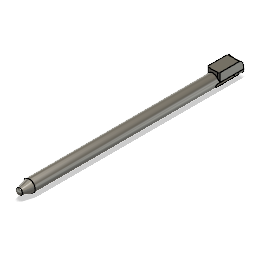
DSi Stylus v9 (Autodesk Fusion 360 design; units mm, degrees)
Autodesk Fusion 360 part; units mm, degrees
sketch "Sketch1" plane through (0, 0, 0) normal (0, 0, 1) x (1, 0, 0)
  circle A0 centre (0, 0) radius 2.5
  dimension "d1" = 5
  constraint coincident A0.centre origin
  measures "d1" diameter of A0
extrude "Extrude1" add sketch "Sketch1" along normal blind 92.2
chamfer "Chamfer1" distance 1.5 distance2 5 1 edges at (-2.3308, -0.904, 92.2) measured on face at (-0.8863, 0.2321, 92.2)
fillet "Fillet1" radius 1.3435 1 edges at (-0.9323, 0.3616, 92.2)
sketch "Sketch2" plane through (0, 0, 0) normal (1, 0, 0) x (0, 0, -1)
  line L0 (0, 0) -> (0, 3.6)
  line L1 (0, 3.6) -> (-10.8, 3.6)
  line L2 (-10.8, 3.6) -> (-10.8, 0)
  line L3 (-10.8, 0) -> (0, 0)
  line L4 (0, 0) -> (0, 3.6)
  dimension "d7" = 3.6
  dimension "d8" = 10.8
  constraint coincident L0.start L3.end
  constraint vertical L0
  constraint horizontal L1
  constraint vertical L2
  constraint horizontal L3
  constraint vertical L4
  measures "d7" distance of L0.start L0.end
  measures "d8" distance of L0.end L1.end
extrude "Extrude2" add sketch "Sketch2" along normal blind 2.5 and the other way blind 2.5
fillet "Fillet2" radius 0.5 1 edges at (2.5, 1.8, 10.8)
fillet "Fillet3" radius 0.5 1 edges at (-2.5, 1.8, 10.8)
sketch "Sketch3" plane through (-2.5, 0, 0) normal (-1, 0, 0) x (0, 0, 1)
  line L0 (10.3, 0) -> (10.3, 3.6)
  line L1 (10.3, 3.6) -> (0, 3.6)
  line L2 (0, 3.6) -> (0, 0)
  line L3 (0, 0) -> (10.3, 0)
  line L4 (0, 3.6) -> (0, 1.6)
  line L5 (0, 1.6) -> (0.6, 1.6)
  line L6 (0.6, 1.6) -> (3.1, 1.6)
  line L7 (3.1, 1.6) -> (3.1, 3.6)
  line L8 (3.1, 3.6) -> (0.6, 3.6)
  line L9 (0.6, 3.6) -> (0.6, 1.6)
  arc A0 (3.1, 3.6) -> (0.6, 1.6) centre (2.65, 1.6) ccw
  line L10 (0, 3.6) -> (0, -2.5)
  line L11 (0, -2.5) -> (0.6202, 1.887)
  dimension "d15" = 2
  dimension "d16" = 0.6
  dimension "d17" = 2.5
  dimension "d18" = 2
  dimension "d19" = 6.1
  constraint coincident L1.end L2.start
  constraint perpendicular L1 L4
  constraint perpendicular L4 L5
  constraint horizontal L6
  constraint vertical L7
  constraint horizontal L8
  constraint vertical L9
  constraint tangent L9 A0
  constraint perpendicular L1 L10
  constraint coincident A0 L11.end
  constraint tangent A0 L11
  measures "d15" distance of L1.end L4.end
  measures "d16" distance of L4.end L5.end
  measures "d17" distance of L5.end L6.end
  measures "d18" distance of L5.end L8.end
  measures "d19" distance of L1.end L10.end
extrude "Extrude3" cut sketch "Sketch3" against normal blind 6.6 contours L3 L10 L11 | L2 L3 L5 L10 L11 | L1 L2 L4 L5 L9 L10 L11 | L1 L8 L9 A0 L11
sketch "Sketch4" plane through (0, 0, 0) normal (1, 0, 0) x (0, 0, -1)
  line L0 (0, 0) -> (-7.9, 0)
  line L1 (-7.9, 0) -> (-7.9, -2.5)
  line L2 (-7.9, -2.5) -> (-6.65, -2.5)
  ellipse E0 centre (-7.275, -2.5) end of major axis (-6.65, -2.5) minor radius 0.5
  line L3 (-7.9, -2.5) -> (-6.65, -2.5) construction
  line L4 (-7.275, -3) -> (-7.275, -2) construction
  dimension "d22" = 7.9
  dimension "d23" = 1.25
  dimension "d24" = 1
  constraint coincident L0.start origin
  constraint horizontal L0
  constraint perpendicular L0 L1
  constraint perpendicular L1 L2
  constraint midpoint L2 E0.centre
  constraint parallel L2 L3
  constraint coincident L1.end E0
  constraint coincident E0 L4.start
  constraint coincident E0 L4.end
  measures "d22" distance of L0.start L0.end
  measures "d23" distance of L1.end L2.end
extrude "Extrude4" add sketch "Sketch4" along normal blind 0.75 and the other way blind 0.75
sketch "Sketch5" plane through (0, 0, 0) normal (1, 0, 0) x (0, 0, -1)
  line L0 (0, 0) -> (-7.9, 0)
  line L1 (-7.9, 0) -> (-6.65, 0)
  line L2 (-7.275, -2.5) -> (-7.275, -1.5)
  line L3 (-7.275, -1.5) -> (-7.275, 0)
  line L4 (-7.275, -0.75) -> (-3.275, -0.75)
  line L5 (-7.275, -0.75) -> (-11.275, -0.75)
  line L6 (-3.275, 0) -> (-11.275, 0)
  arc A0 (-11.275, 0) -> (-11.275, -1.5) centre (-11.275, -0.75) ccw
  line L7 (-11.275, -1.5) -> (-3.275, -1.5)
  arc A1 (-3.275, -1.5) -> (-3.275, 0) centre (-3.275, -0.75) ccw
  line L8 (-3.275, -0.75) -> (-11.275, -0.75) construction
  dimension "d29" = 7.9
  dimension "d30" = 1.25
  dimension "d32" = 1
  dimension "d33" = 4
  dimension "d34" = 4
  constraint coincident L0.start origin
  constraint horizontal L0
  constraint parallel L0 L1
  constraint midpoint L1 L3.end
  constraint perpendicular L0 L3
  constraint midpoint L3 L4.start
  constraint perpendicular L3 L4
  constraint perpendicular L3 L5
  constraint tangent L6 A0
  constraint tangent A0 L7
  constraint parallel L6 L7
  constraint tangent L7 A1
  constraint tangent L6 A1
  constraint coincident L5.end A0.centre
  constraint perpendicular L3 L8
  constraint coincident L4.end A1.centre
  measures "d29" distance of L0.start L0.end
  measures "d30" distance of L0.end L1.end
  measures "d32" distance of L2.start L2.end
  measures "d33" distance of L4.start L4.end
  measures "d34" distance of L4.start L5.end
extrude "Extrude5" cut sketch "Sketch5" along normal blind 9.6 and the other way blind 13.9
moveface "MoveFace1" [suppressed]
move_face "OffsetFaces1" [suppressed]
sketch "Sketch6" plane through (0, 0, 0) normal (0, 0, 1) x (1, 0, 0)
  line L0 (0, 0) -> (0, -2.5)
  line L1 (0, -2.5) -> (0, -3)
  line L2 (0, -3) -> (0.75, -3)
  circle A0 centre (0, 0) radius 2.4
  line L3 (0.75, -3) -> (0.75, -2.2798)
  line L4 (0.4792, -3) -> (1.7521, -1.6401)
  dimension "d39" = 0.75
  dimension "d42" = 4.8
  constraint coincident L0.start A0.centre
  constraint vertical L0
  constraint parallel L0 L1
  constraint perpendicular L1 L2
  constraint coincident A0 L3.end
  constraint perpendicular L2 L3
  constraint coincident L2 L4.start
  constraint coincident A0 L4.end
  constraint tangent A0 L4
  measures "d39" distance of L1.end L2.end
  measures "d42" diameter of A0
move_body "Move2" [suppressed]
sketch "Sketch7" plane through (0, 0, 0) normal (0.730162, -0.683274, 0) x (0, 0, -1)
  line L0 (-10.3, 2.4) -> (-11.275, 2.4)
  line L1 (-11.275, 2.4) -> (-11.275, -2.4)
  line L2 (-11.275, -2.4) -> (-10.3, -2.4)
  line L3 (-10.3, -2.4) -> (-3.275, -2.4)
  line L4 (-3.275, -2.4) -> (-3.275, 2.4)
  line L5 (-3.275, 2.4) -> (-10.3, 2.4)
  line L6 (-11.275, -2.4) -> (-3.275, -2.4) construction
  line L7 (-3.275, -2.4) -> (-3.275, 2.4) construction
  line L8 (-3.275, 2.4) -> (-11.275, 2.4) construction
  line L9 (-11.275, 2.4) -> (-11.275, -2.4) construction
extrude "Extrude6" [suppressed]
equation "d7 = 2.5 mm + 1.1 mm"
equation "d19 = 3.6 mm + 2.5 mm"
named bodies: "DSi Stylus"
